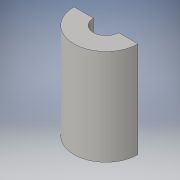
# Autodesk Inventor part: Linear Actuatur piece 2
Saved by Autodesk Inventor 2016 (Build 200138000, 138)
## iProperties
Created: 2015-12-05
Part Number: Linear Actuatur piece 2
Material: Generic
Document SubType Name: Modeling
Designer: Javier
Density: 1 g/cm^3
Appearance: Default
Author: Javier
Autodesk Inventor part; units mm, degrees
ref_plane "YZ Plane" through (0, 0, 0) normal (1, 0, 0) x (0, 1, 0)
ref_plane "XZ Plane" through (0, 0, 0) normal (0, 1, 0) x (-1, 0, 0)
ref_plane "XY Plane" through (0, 0, 0) normal (0, 0, 1) x (1, 0, 0)
sketch "Sketch1" plane through (0, 0, 0) normal (0, 1, 0) x (-1, 0, 0)
  circle A0 centre (0, 0) radius 25.4
  circle A1 centre (0, 0) radius 10
  line L0 (-25.4, 0) -> (-10, 0)
  line L1 (10, 0) -> (25.4, 0)
  dimension "d0" = 50.8
  dimension "d1" = 20
  constraints: 4 end point, 4 point on circle, 2 centre point, 2 coincident, 2 point on line, 1 horizontal
  measures "d0" diameter of A0
  measures "d1" diameter of A1
extrude "Extrusion1" add sketch "Sketch1" along normal mid plane 76.2 contours L1 A1 L0 A0 picked at (-20.0206, 2.0262)
sketch "Sketch2" plane through (0, 0, 0) normal (0, 0, 1) x (1, 0, 0)
  circle A0 centre (0, -6) radius 3.25
  line L0 (46.8316, 0) -> (-44.45, 0)
  point P0 (0, 0)
  dimension "d4" = 6.5
  dimension "d6" = 6
  constraints: 2 end point, 1 centre point, 1 horizontal
  measures "d4" diameter of A0
  measures "d6" distance from line of A0.centre L0
extrude "Extrusion2" cut sketch "Sketch2" along normal blind 11
body "Solid1"
